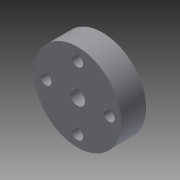
# Autodesk Inventor part: Hub
Saved by Autodesk Inventor 2015 (Build 190159000, 159)
## iProperties
Created: 2016-10-18
Part Number: Hub
Material: Generic
Document SubType Name: Modeling
Designer: James Yelland
Density: 1 g/cm^3
Appearance: Default
Author: James Yelland
Autodesk Inventor part; units mm, degrees
ref_plane "YZ Plane" through (0, 0, 0) normal (1, 0, 0) x (0, 1, 0)
ref_plane "XZ Plane" through (0, 0, 0) normal (0, 1, 0) x (-1, 0, 0)
ref_plane "XY Plane" through (0, 0, 0) normal (0, 0, 1) x (1, 0, 0)
sketch "Sketch1" plane through (0, 0, 0) normal (0, 1, 0) x (-1, 0, 0)
  circle A0 centre (0, 0) radius 8.75
  circle A1 centre (0, 0) radius 1.5
  line L0 (0, 0) -> (6.35, 0)
  circle A2 centre (6.35, 0) radius 1.1
  circle A3 centre (0, 6.35) radius 1.1
  circle A4 centre (-6.35, 0) radius 1.1
  circle A5 centre (0, -6.35) radius 1.1
  dimension "d0" = 17.5
  dimension "d1" = 3
  dimension "d2" = 6.35
  dimension "d3" = 2.2
  dimension "d6" = 360
  constraints: 6 centre point, 3 coincident, 2 end point, 1 horizontal, 9 other
  measures "d0" diameter of A0
  measures "d1" diameter of A1
  measures "d2" distance of L0.start L0.end
  measures "d3" diameter of A2
extrude "Extrusion1" add sketch "Sketch1" along normal blind 5
body "Solid1"
